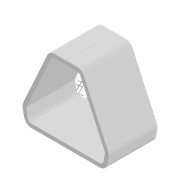
# Autodesk Inventor part: ShoulderChestBracket
Saved by Autodesk Inventor 2020 (Build 240168000, 168)
## iProperties
Created: 2020-04-01
Part Number: ShoulderChestBracket
Material: Generic
Document SubType Name: Sheet Metal
Designer: valer
Density: 1 g/cm^3
Sheet Metal Rule: Default
Appearance: Default
Author: valer
Autodesk Inventor part; units mm, degrees
ref_plane "YZ Plane" through (0, 0, 0) normal (1, 0, 0) x (0, 1, 0)
ref_plane "XZ Plane" through (0, 0, 0) normal (0, 1, 0) x (-1, 0, 0)
ref_plane "XY Plane" through (0, 0, 0) normal (0, 0, 1) x (1, 0, 0)
sketch "Outline" plane through (0, 0, 0) normal (0, 0, 1) x (1, 0, 0)
  line L0 (0, 59.2667) -> (0, 0) construction
  line L1 (0, 0) -> (31.75, 0)
  line L2 (31.75, 0) -> (33.9553, 12.5071)
  line L3 (33.9553, 12.5071) -> (12.7, 59.2667)
  line L4 (12.7, 59.2667) -> (0.254, 59.2667)
  line L5 (-12.7, 59.2667) -> (0, 59.2667)
  line L6 (-33.9553, 12.5071) -> (-12.7, 59.2667)
  line L7 (-31.75, 0) -> (-33.9553, 12.5071)
  line L8 (0, 0) -> (-31.75, 0)
  line L9 (6.35, 59.2667) -> (6.35, 0) construction
  line L10 (12.7, 59.2667) -> (12.7, 0) construction
  line L11 (6.35, 0) -> (12.7, 0)
  line L12 (9.525, 0) -> (9.525, 59.2667) construction
  line L13 (29.4386, 52.925) -> (40.2933, 29.0458) construction
  line L14 (40.2933, 29.0458) -> (16.8349, 18.3824) construction
  line L15 (16.8349, 18.3824) -> (5.9802, 42.2616) construction
  line L16 (5.9802, 42.2616) -> (29.4386, 52.925) construction
  line L17 (34.866, 40.9854) -> (11.4075, 30.322) construction
  line L18 (33.2893, 44.4539) -> (9.8309, 33.7905) construction
  line L19 (36.4426, 37.5169) -> (12.9842, 26.8535) construction
  line L20 (0.254, 55.5625) -> (0, 55.5625)
  dimension "d0" = 31.75
  dimension "d1" = 100
  dimension "d2" = 12.7
  dimension "d3" = 12.7
  dimension "d4" = 59.2667
  dimension "d5" = 3.81
  dimension "d6" = 12.7
  dimension "d7" = 0.254
  measures "d0" distance of L0.end L1.end
  measures "d1" angle of L2 L1
  measures "d2" distance of L1.end L2.end
  measures "d3" distance of L0.start L3.end
  measures "d4" distance of L0.start L0.end
  measures "d5" distance between parallel lines of L17 L18
  measures "d6" distance from line of L3.end L16
  measures "d7" distance of L4.end L0.start
contour flange "Contour Flange1" sketch "Outline" thickness 3.048 bend radius 3.048 width 38.1 along (0, 0, 1) mid plane no both sides no wall seen from (6.477, 59.2667, 0) lies toward (0, -1, 0) curves L4 L3 L2 L1 L8 L7 L6 L5
bend "Bend1"
corner "Corner1"
equation "\"d9\" = Thickness"
equation "\"d10\" = BendReliefWidth"
equation "\"d11\" = BendReliefDepth"
equation "\"d12\" = MinimumRemnant"
equation "\"d13\" = TransitionRadius"
equation "\"d15\" = BendRadius"
equation "\"d17\" = CornerReliefSize"
equation "\"d18\" = GapSize"
equation "\"d19\" = JacobiRadiusSize"
equation "\"BendRadius\" = Thickness"
equation "\"BendReliefWidth\" = Thickness"
equation "\"BendReliefDepth\" = 0.5 * Thickness"
equation "\"CornerReliefSize\" = 4 * Thickness"
equation "\"MinimumRemnant\" = 2 * Thickness"
equation "\"TransitionRadius\" = BendRadius"
equation "\"JacobiRadiusSize\" = BendRadius"
equation "\"GapSize\" = Thickness"
equation "\"Thickness\" = 3.048"
body "Solid1"
